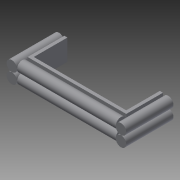
# Autodesk Inventor part: Bumper
Saved by Autodesk Inventor 2014 SP1 (Build 180222100, 222)
## iProperties
Created: 2014-01-18
Part Number: Bumper
Material: Generic
Document SubType Name: Modeling
Designer: Paul
Density: 1 g/cm^3
Appearance: Default
Author: Paul
Autodesk Inventor part; units mm, degrees
ref_plane "YZ Plane" through (0, 0, 0) normal (1, 0, 0) x (0, 1, 0)
ref_plane "XZ Plane" through (0, 0, 0) normal (0, 1, 0) x (-1, 0, 0)
ref_plane "XY Plane" through (0, 0, 0) normal (0, 0, 1) x (1, 0, 0)
sketch "Sketch1" plane through (0, 0, 0) normal (0, 0, 1) x (1, 0, 0)
  line L0 (0, 0) -> (596.9, 0)
  line L1 (596.9, 0) -> (596.9, 127)
  line L2 (596.9, 127) -> (0, 127)
  line L3 (0, 127) -> (0, 0)
  dimension "d0" = 127
  dimension "d1" = 596.9
  constraints: 8 end point, 2 parallel, 1 horizontal, 1 perpendicular
  measures "d0" distance of L2.end L0.start
  measures "d1" distance between parallel lines of L1 L3
extrude "Extrusion1" add sketch "Sketch1" along normal blind 19.05
sketch "Sketch2" plane through (0, 0, 0) normal (0, 0, -1) x (-1, 0, 0)
  line L0 (0, 0) -> (-596.9, 0) projected
  line L1 (-596.9, 127) -> (0, 127) projected
  line L2 (-596.9, 0) -> (-596.9, 127) projected
  line L3 (-596.9, 127) -> (-577.85, 127)
  line L4 (-577.85, 127) -> (-577.85, 0)
  line L5 (-577.85, 0) -> (-596.9, 0)
  line L6 (-596.9, 0) -> (-596.9, 127)
  line L7 (0, 0) -> (-19.05, 0)
  line L8 (-19.05, 0) -> (-19.05, 127)
  line L9 (-19.05, 127) -> (0, 127)
  line L10 (0, 127) -> (0, 0)
  dimension "d4" = 19.05
  dimension "d5" = 19.05
  constraints: 16 end point, 4 parallel, 2 horizontal, 2 perpendicular, 2 point on line
  measures "d4" distance between parallel lines of L10 L8
  measures "d5" distance between parallel lines of L2 L4
extrude "Extrusion2" add sketch "Sketch2" along normal blind 203.2 contours L0 L8 L1 L10 | L0 L2 L1 L4
sketch "Sketch3" plane through (596.9, 0, 19.05) normal (1, 0, 0) x (0, 0, -1)
  line L0 (222.25, 127) -> (0, 127) projected
  line L1 (0, 0) -> (0, 127) projected
  circle A0 centre (-31.75, 95.25) radius 31.75
  circle A1 centre (-31.75, 31.75) radius 31.75
  point P0 (19.05, 0)
  dimension "d8" = 63.5
  dimension "d9" = 63.5
  dimension "d10" = 31.75
  dimension "d11" = 31.75
  dimension "d12" = 31.75
  constraints: 2 centre point, 1 equal radius
  measures "d8" diameter of A0
  measures "d9" diameter of A1
  measures "d10" distance from line of L1 A1.centre
  measures "d11" distance from line of L1 A0.centre
  measures "d12" distance from line of L0 A0.centre
extrude "Extrusion3" add sketch "Sketch3" against normal blind 596.9 contours A1 | A0
sketch "Sketch4" plane through (0, 0, -203.2) normal (0, 0, -1) x (-1, 0, 0)
  line L0 (-577.85, 127) -> (-596.9, 127) projected
  circle A0 centre (-628.65, 95.25) radius 31.75
  circle A1 centre (-628.65, 31.75) radius 31.75
  circle A2 centre (31.75, 95.25) radius 31.75
  circle A3 centre (31.75, 31.75) radius 31.75
  line L1 (0, 0) -> (0, 127) projected
  line L2 (0, 127) -> (-19.05, 127) projected
  dimension "d15" = 63.5
  dimension "d16" = 63.5
  dimension "d17" = 660.4
  dimension "d18" = 31.75
  dimension "d19" = 31.75
  constraints: 4 centre point, 4 tangent, 2 equal radius
  measures "d15" diameter of A2
  measures "d16" diameter of A0
  measures "d17" distance of A0.centre A2.centre
  measures "d18" distance from line of L0 A0.centre
  measures "d19" distance from line of L2 A2.centre
extrude "Extrusion4" add sketch "Sketch4" against normal blind 285.75 contours A0 | A1 | A2 | A3
body "Solid1"
